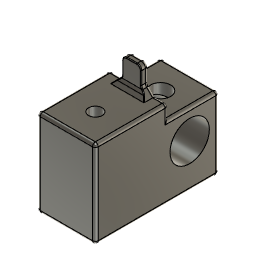
PoleOSSMUlanzi_v6 (Autodesk Fusion 360 design; units mm, degrees)
Autodesk Fusion 360 part; units mm, degrees
note: some values were not read from the file. Set by a fixed rule: which sketch regions a step uses.
sketch "Sketch1" plane through (0, 0, 0) normal (1, 0, 0) x (0, 1, 0)
  circle A0 centre (0, 0) radius 13.55
  line L0 (20, -30) -> (-20, -30)
  line L1 (-20, -30) -> (-20, 20)
  line L2 (-20, 20) -> (20, 20)
  line L3 (20, 20) -> (20, -30)
  point P0 (0, -13.55)
  dimension "d1" = 27.1
  dimension "d2" = 40
  dimension "d12" = 16.45
  dimension "d45" = 20
  dimension "d46" = 30
  dimension "d47" = 20
  constraint coincident A0.centre origin
  constraint horizontal L0
  constraint perpendicular L0 L1
  constraint parallel L0 L2
  constraint parallel L1 L3
  constraint coincident A0 P0
  constraint vertical A0.centre P0
  measures "d1" diameter of A0
  measures "d2" distance of L1.end L2.end
  measures "d12" distance of L0 P0
  measures "d45" distance of L2 A0.centre
  measures "d46" distance of A0.centre L0
  measures "d47" distance of A0.centre L1
extrude "Extrude1" add sketch "Sketch1" against normal blind 40
sketch "Sketch2" plane through (0, 0, 20) normal (0, 0, 1) x (-1, 0, 0)
  line L0 (0, 20) -> (0, -20)
  line L1 (0, -20) -> (40, -20)
  line L2 (40, -20) -> (40, 20)
  line L3 (40, 20) -> (0, 20)
  circle A0 centre (20, 0) radius 3.75
  line L4 (40, 0) -> (0, 0) construction
  circle A1 centre (20, 0) radius 6.9
  dimension "d6" = 7.5
  dimension "d9" = 20
  dimension "d17" = 13.8
  dimension "d80" = 20
  constraint midpoint L2 L4.start
  constraint coincident L4.end origin
  constraint coincident A0.centre L4
  constraint concentric A0 A1
  measures "d6" diameter of A0
  measures "d9" distance of A0.centre L4.start
  measures "d17" diameter of A1
  measures "d80" distance of L0 A0.centre
extrude "Extrude2" cut sketch "Sketch2" against normal up to surface (50 mm away) contours A0
extrude "Extrude4" cut sketch "Sketch2" against normal blind 13 contours A1
sketch "Sketch3" plane through (0, 0, -30) normal (0, 0, -1) x (1, 0, 0)
  circle A0 centre (-20, 0) radius 3.75
  line L0 (0, -20) -> (0, 20)
  line L1 (0, 20) -> (-40, 20)
  line L2 (-40, 20) -> (-40, -20)
  line L3 (-40, -20) -> (0, -20)
  circle A1 centre (-20, 0) radius 3.75
  line L4 (-23.7239, 6.45) -> (-27.4478, 0)
  line L5 (-27.4478, 0) -> (-23.7239, -6.45)
  line L6 (-23.7239, -6.45) -> (-16.2761, -6.45)
  line L7 (-16.2761, -6.45) -> (-12.5522, 0)
  line L8 (-12.5522, 0) -> (-16.2761, 6.45)
  line L9 (-16.2761, 6.45) -> (-23.7239, 6.45)
  point P0 (-20, 0)
  dimension "d14" = 6.45
  constraint coincident P0 A0.centre
  constraint horizontal L9
  measures "d14" distance of P0 L9
extrude "Extrude3" cut sketch "Sketch3" against normal blind 6.5 contours L4 L5 L6 L7 L8 L9
sketch "Sketch4" plane through (-40, 0, 0) normal (-1, 0, 0) x (0, -1, 0)
  circle A0 centre (0, 0) radius 13.55
  line L0 (20, 20) -> (-20, 20)
  line L1 (-20, 20) -> (-20, -30)
  line L2 (-20, -30) -> (20, -30)
  line L3 (20, -30) -> (20, 20)
  circle A1 centre (0, 0) radius 13.55
  line L4 (20, -30) -> (-28, -30)
  line L5 (-28, -30) -> (-28, 20)
  line L6 (-28, 20) -> (20, 20)
  line L7 (20, 20) -> (20, -30)
  circle A2 centre (0, 0) radius 4.5
  dimension "d22" = 50
  dimension "d25" = 9
  dimension "d41" = 20
  dimension "d42" = 28
  dimension "d48" = 50
  constraint horizontal L4
  constraint perpendicular L4 L5
  constraint parallel L4 L6
  constraint parallel L5 L7
  constraint coincident A0.centre A1.centre
  constraint collinear L0 L6
  measures "d22" distance of L4.end L5.end
  measures "d25" diameter of A2
  measures "d41" distance of L7 A0.centre
  measures "d42" distance of L5 A0.centre
  measures "d48" distance of L0.end L1.end
ref_plane "WorkPlane1" through (-20, 0, 30) normal (0, 0, 1) x (0, 1, 0)
sketch "Sketch8" plane through (0, 0, 30) normal (0, 0, 1) x (-1, 0, 0)
  circle A0 centre (20, 0) radius 6.9
  line L0 (0, 20) -> (0, -20)
  line L1 (0, -20) -> (40, -20)
  line L2 (40, -20) -> (40, 20)
  line L3 (40, 20) -> (0, 20)
  line L4 (40, 20) -> (0, 20)
  line L5 (0, 20) -> (0, 65)
  line L6 (0, 65) -> (40, 65)
  line L7 (40, 65) -> (40, 20)
  circle A1 centre (20, 45) radius 4.675
  line L8 (13.5, 15) -> (26.5, 15)
  line L9 (26.5, 15) -> (26.5, 20)
  line L10 (26.5, 20) -> (13.5, 20)
  line L11 (13.5, 20) -> (13.5, 15)
  point P0 (20, 20)
  point P1 (20, 20)
  dimension "d83" = 9.35
  dimension "d84" = 20
  dimension "d85" = 20
  dimension "d86" = 20
  dimension "d87" = 25
  dimension "d88" = 13
  dimension "d89" = 5
  constraint horizontal L4
  constraint vertical L5
  constraint horizontal L6
  constraint vertical L7
  constraint coincident L2.end L3.start
  constraint horizontal L8
  constraint vertical L9
  constraint horizontal L10
  constraint vertical L11
  constraint midpoint L10 P1
  constraint midpoint L4 P1
  constraint coincident P1 P0
  measures "d83" diameter of A1
  measures "d84" distance of L5 A1.centre
  measures "d85" distance of L7 A1.centre
  measures "d86" distance of L6 A1.centre
  measures "d87" distance of L4 A1.centre
  measures "d88" distance of L8.start L8.end
  measures "d89" distance of L8.start L10.end
extrude "Extrude9" add sketch "Sketch8" along normal blind 18 and the other way up to surface (10 mm away) contours L3 L4 L8 L9 L10 L11
extrude "Extrude10" add sketch "Sketch8" against normal blind 60 contours L3 L4 L5 L6 L7 L10
extrude "Extrude11" add 2 faces at (-9, -20, 26.6667) (-35.5, -20, 26.6667) along direction (0, 1, 0) up to surface end surface through (-13.5, -15, 30) normal (0, 1, 0) offset 0
chamfer "Chamfer5" distance 5 angle 45 2 edges at (-13.5, -17.5, 30) (-26.5, -17.5, 30)
sketch "Sketch9" plane through (0, -15, 0) normal (0, 1, 0) x (-1, 0, 0)
  line L0 (26.5, 35) -> (26.5, 48)
  line L1 (26.5, 48) -> (13.5, 48)
  line L2 (13.5, 48) -> (13.5, 35)
  line L3 (13.5, 35) -> (8.5, 30)
  line L4 (8.5, 30) -> (0, 30)
  line L5 (0, 30) -> (0, 20)
  line L6 (0, 20) -> (40, 20)
  line L7 (40, 20) -> (40, 30)
  line L8 (40, 30) -> (31.5, 30)
  line L9 (31.5, 30) -> (26.5, 35)
  line L10 (13.5, 35) -> (26.5, 35)
  line L11 (31.5, 30) -> (8.5, 30)
  line L12 (26.5, 35) -> (31.5, 30)
  line L13 (8.5, 30) -> (13.5, 35)
  constraint coincident L2.end L3.start
  constraint coincident L0.start L9.end
  constraint coincident L8.end L9.start
  constraint coincident L3.end L4.start
fillet "Fillet10" radius 2 16 edges at (-40, -40, 30) (-40, 2.5, 20) (-40, -22.5, -30) (-40, -22.5, -30) (-40, -65, 0) (-20, -65, 30) (-20, -65, -30) (0, -65, 0) (0, -22.5, -30) (0, -22.5, -30) (0, 20, -5) (-20, 20, 20) (0, -40, 30) (0, 2.5, 20) (-40, 20, -5) (-20, 20, -30)
fillet "Fillet10" radius 2 7 edges at (-35.75, -15, 30) (-4.25, -15, 30) (-29, -15, 32.5) (-11, -15, 32.5) (-13.5, -15, 41.5) (-26.5, -15, 41.5) (-20, -15, 48)
fillet "Fillet10" radius 2 2 edges at (-40, -15, 25) (0, -15, 25)
chamfer "Chamfer7" distance 3 angle 45 1 edges at (-20, -20, 30)
fillet "Fillet11" radius 3 2 edges at (-26.5, -18.5, 35) (-13.5, -18.5, 35)
fillet "Fillet11" radius 3 2 edges at (-13.5, -17.5, 48) (-26.5, -17.5, 48)
fillet "Fillet13" radius 3 1 edges at (-20, -20, 33)
fillet "Fillet12" radius 0.5 13 edges at (-13.5, -20, 40.6213) (-13.3025, -20, 35.1722) (-12.6796, -20.0006, 34.1812) (-11.5388, -20.2521, 33.0388) (-9.5607, -21.9393, 31.0607) (-14.3787, -20, 47.1213) (-20, -20, 48) (-25.6213, -20, 47.1213) (-26.5, -20, 40.6213) (-26.6975, -20, 35.1722) (-27.3204, -20.0006, 34.1812) (-28.4612, -20.2521, 33.0388) (-30.4393, -21.9393, 31.0607)
sketch "Sketch10" plane through (0, 0, -30) normal (0, 0, -1) x (1, 0, 0)
  line L0 (-27.4478, 0) -> (-23.7239, 6.45)
  line L1 (-23.7239, 6.45) -> (-16.2761, 6.45)
  line L2 (-16.2761, 6.45) -> (-12.5522, 0)
  line L3 (-12.5522, 0) -> (-16.2761, -6.45)
  line L4 (-16.2761, -6.45) -> (-23.7239, -6.45)
  line L5 (-23.7239, -6.45) -> (-27.4478, 0)
  circle A0 centre (-20, 45) radius 4.675
  line L6 (-38, -18) -> (-2, -18)
  line L7 (-2, -18) -> (-2, 63)
  line L8 (-2, 63) -> (-38, 63)
  line L9 (-38, 63) -> (-38, -18)
  circle A1 centre (-20, 45) radius 4.675
  circle A2 centre (-20, 45) radius 7.125
  dimension "d130" = 14.25
  constraint concentric A0 A2
  measures "d130" diameter of A2
extrude "Extrude13" cut sketch "Sketch10" against normal blind 10.5 contours A2
equation "d14 = ( 12.9 / 2 ) * 1 mm"
equation "d22 = d48"
